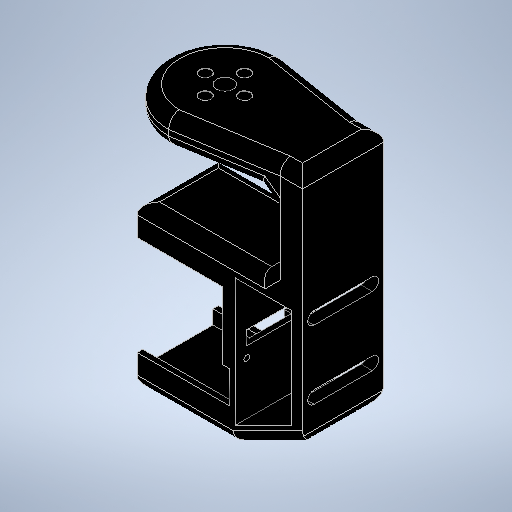
# Autodesk Inventor part: wahaczv6
Saved by Autodesk Inventor 2025.3 (Build 293356000, 356)
## iProperties
Created: 2026-04-05
Part Number: wahaczv6
Material: PCTG 20%
Document SubType Name: Modeling
Designer: ksawe
Density: 1.541 g/cm^3
Appearance: Anodized - Black
Mass: 108.544 g
Surface Area: 247.96 cm^2
Volume: 70.4373 cm^3
Author: ksawe
Autodesk Inventor part; units mm, degrees
ref_plane "YZ Plane" through (0, 0, 0) normal (1, 0, 0) x (0, 1, 0)
ref_plane "XZ Plane" through (0, 0, 0) normal (0, 1, 0) x (-1, 0, 0)
sketch "Sketch1" plane through (0, 0, 0) normal (0, 0, 1) x (1, 0, 0)
  line L0 (-59, 0) -> (-59, 6)
  line L1 (-59, 6) -> (-26, 6)
  line L2 (-26, 6) -> (-26, 51.5)
  line L3 (-26, 51.5) -> (-59, 51.5)
  line L4 (-59, 51.5) -> (-59, 57.5)
  line L5 (-59, 57.5) -> (-8, 57.5)
  line L6 (-8, 57.5) -> (-8, 95)
  line L7 (-8, 95) -> (0, 95)
  line L8 (-24, 51.5) -> (-4, 51.5)
  line L9 (-24, 51.5) -> (-24, 16)
  line L10 (-4, 51.5) -> (-4, 16)
  line L11 (-4, 16) -> (-24, 6)
  line L12 (-59, 0) -> (-24, 0)
  line L13 (-24, 0) -> (0, 12)
  line L14 (-24, 16) -> (-24, 6)
  line L15 (0, 95) -> (0, 12)
  point P0 (0, 0)
  dimension "d1" = 33
  dimension "d3" = 33
  dimension "d4" = 6
  dimension "d5" = 6
  dimension "d6" = 51
  dimension "d8" = 8
  dimension "d9" = 95
  dimension "d13" = 2
  dimension "d116" = 12
  dimension "d117" = 4
  dimension "d118" = 57.5
  constraints: 32 end point, 7 vertical, 5 vertical alignment, 4 horizontal, 4 horizontal alignment, 2 parallel, 2 perpendicular, 2 point on line
  measures "d1" distance of L0.end L1.end
  measures "d3" distance of L2.end L3.end
  measures "d4" distance of L3.end L4.end
  measures "d5" distance of L0.start L0.end
  measures "d6" distance of L4.end L5.end
  measures "d8" distance of L6.end L7.end
  measures "d9" distance of L7.end point (0, 0)
  measures "d13" distance between parallel lines of L9 L2
  measures "d116" vertical distance of L13.end L12.end
  measures "d117" distance between parallel lines of L15 L10
  measures "d118" distance between parallel lines of L12 L5
extrude "Extrusion1" add sketch "Sketch1" along normal mid plane 29
sketch "Sketch2" plane through (-8, 95, 14.5) normal (0, 1, 0) x (1, 0, 0)
  line L0 (0, 29) -> (0, 0) projected
  arc A0 (-34.2, 34.5) -> (-34.2, -5.5) centre (-34.2, 14.5) ccw
  line L1 (4, 29) -> (4, 0) projected
  line L2 (-34.2, 34.5) -> (0, 29)
  line L3 (8, 0) -> (0, 0) projected
  line L4 (0, 0) -> (-34.2, -5.5)
  circle A1 centre (-34.2, 14.5) radius 3
  circle A2 centre (-34.2, 21.5) radius 1.25
  circle A3 centre (-41.2, 14.5) radius 1.25
  circle A4 centre (-34.2, 7.5) radius 1.25
  circle A5 centre (-27.2, 14.5) radius 1.25
  point P0 (8, 14.5)
  point P1 (0, 14.5)
  point P2 (0, 14.5)
  dimension "d17" = 40
  dimension "d18" = 34.2
  dimension "d47" = 6
  dimension "d51" = 360
  dimension "d53" = 7
  dimension "d54" = 2.5
  constraints: 6 centre point, 4 end point, 2 midpoint, 2 point on circle, 2 vertical alignment, 1 coincident, 1 equal length, 1 horizontal alignment, 10 other
  measures "d17" diameter of A0
  measures "d18" distance of point (0, 14.5) A0.centre
  measures "d47" diameter of A1
  measures "d53" horizontal distance of A5.centre A2.centre
  measures "d54" diameter of A2
extrude "Extrusion2" add sketch "Sketch2" against normal blind 10 contours L0 L4 A0 L2 | A2 | A3 | A4 | A5
sketch "Sketch3" plane through (-26, 6, 14.5) normal (-1, 0, 0) x (0, 0, 1)
  line L0 (-29, 45.5) -> (0, 45.5) projected
  line L1 (-29, 0) -> (-29, 45.5) projected
  line L2 (0, 45.5) -> (0, 0) projected
  line L3 (-29, 0) -> (0, 0) construction
  line L4 (-14.5, 0) -> (-14.5, 45.5)
  line L5 (-29, 45.5) -> (0, 45.5) projected
  line L6 (-24.5, 40.5) -> (-4.5, 40.5)
  line L7 (-25.1, 27.5) -> (-3.9, 27.5)
  line L8 (-29, 45.5) -> (0, 45.5) construction
  line L9 (-25.1, 27.5) -> (-25.1, 22.5)
  line L10 (-25.1, 22.5) -> (-26.1, 22.5)
  line L11 (-26.1, 22.5) -> (-26.1, 27.5)
  line L12 (-26.1, 27.5) -> (-25.1, 27.5)
  line L13 (-3.9, 27.5) -> (-3.9, 22.5)
  line L14 (-3.9, 22.5) -> (-2.9, 22.5)
  line L15 (-2.9, 22.5) -> (-2.9, 27.5)
  line L16 (-2.9, 27.5) -> (-3.9, 27.5)
  line L17 (-25.1, 22.5) -> (-3.9, 22.5)
  line L18 (-29, 45.5) -> (-29, 0) projected
  line L19 (-22, 22.5) -> (-22, 20.5)
  line L20 (-24.5, 16.5) -> (-29, 16.5)
  line L21 (-24.5, 40.5) -> (-24.5, 27.5)
  line L22 (-7, 20.5) -> (-4.5, 16.5)
  line L23 (-4.5, 16.5) -> (0, 16.5)
  line L24 (-4.5, 40.5) -> (-4.5, 27.5)
  line L25 (-7, 22.5) -> (-7, 20.5)
  circle A0 centre (-24.89, 43.14) radius 1.05
  circle A1 centre (-24.89, 18.69) radius 1.05
  circle A2 centre (-4.11, 43.14) radius 1.05
  circle A3 centre (-4.11, 18.69) radius 1.05
  line L26 (-22, 20.5) -> (-24.5, 16.5)
  point P0 (-14.5, -6)
  point P1 (-14.5, 40.5)
  point P2 (-14.5, 27.5)
  point P3 (-29, 14)
  point P4 (-14.5, 40.5)
  point P5 (-14.5, 45.5)
  point P6 (-14.5, 27.5)
  point P7 (-14.5, 22.5)
  dimension "d22" = 5
  dimension "d25" = 2
  dimension "d26" = 5
  dimension "d30" = 13
  dimension "d33" = 2.1
  dimension "d34" = 2.1
  dimension "d35" = 24.45
  dimension "d37" = 2.36
  dimension "d40" = 6
  dimension "d44" = 4.11
  dimension "d46" = 2.5
  dimension "d83" = 2.9
  dimension "d84" = 1.6
  dimension "d85" = 1
  dimension "d86" = 20
  constraints: 40 end point, 10 symmetric about line, 6 midpoint, 5 perpendicular, 4 centre point, 4 vertical alignment, 2 horizontal, 2 point on line, 2 vertical, 2 other
  measures "d22" distance between parallel lines of L0 L6
  measures "d25" distance of L19.start L19.end
  measures "d26" distance of L10.end L11.end
  measures "d30" distance of L6.start L21.end
  measures "d33" diameter of A0
  measures "d34" diameter of A1
  measures "d35" distance of A0.centre A1.centre
  measures "d37" distance from line of L0 A0.centre
  measures "d40" distance between parallel lines of L20 L17
  measures "d44" distance from line of L18 A1.centre
  measures "d46" horizontal distance of L19.end L20.start
  measures "d83" distance between parallel lines of L1 L11
  measures "d84" distance from line of L11.end L21
  measures "d85" distance between parallel lines of L9 L11
  measures "d86" distance of L6.start L6.end
extrude "Extrusion3" add sketch "Sketch3" along normal blind 2.5 contours L0 L4 L6 L21 L7 L12 L11 L10 L17 L19 L26 L20 L1 | L0 L2 L23 L22 L25 L17 L14 L15 L16 L7 L24 L6 L4 | L9 L10 L11 L12 | L16 L15 L14 L13
extrude "Extrusion4" cut sketch "Sketch3" against normal up to surface (2 mm away) contours L7 L13 L17 L4 | L4 L17 L9 L7 | A0 | A1 | A2 | A3
hole "Hole1" at (-49.2, 95, 0) at (-42.2, 95, -7) at (-35.2, 95, 0) at (-42.2, 95, 7) direction (0, -1, 0) diameter 4 depth 7 countersink diameter 4.2 countersink angle 90
ref_plane "Work Plane1" through (-26, 28.5, 0) normal (0, 1, 0) x (1, 0, 0)
sketch "Sketch6" plane through (-59, 6, 14.5) normal (0, 1, 0) x (1, 0, 0)
  line L0 (33, 29) -> (33, 0) projected
  line L1 (33, 2) -> (0, 2)
  line L2 (33, 0) -> (0, 0) projected
  line L3 (0, 29) -> (0, 0) projected
  line L4 (33, 27) -> (0, 27)
  line L5 (0, 29) -> (33, 29) projected
  point P0 (59, 14.5)
  dimension "d74" = 2
  dimension "d75" = 2
  constraints: 4 end point, 3 point on line, 1 parallel, 1 perpendicular
  measures "d74" distance between parallel lines of L2 L1
  measures "d75" distance between parallel lines of L5 L4
extrude "Extrusion7" add sketch "Sketch6" along normal blind 5 contours L0 L4 L3 L5 | L0 L2 L3 L1
sketch "Sketch7" plane through (-59, 51.5, -14.5) normal (0, -1, 0) x (1, 0, 0)
  line L0 (0, 0) -> (0, 29) projected
  line L1 (0, 29) -> (30.5, 29) projected
  line L2 (30.5, 0) -> (0, 0) projected
  line L3 (30.5, 0) -> (30.5, 29) projected
  line L4 (30.5, 2) -> (0, 2)
  line L5 (30.5, 27) -> (0, 27)
  point P0 (59, 14.5)
  dimension "d78" = 2
  dimension "d79" = 2
  constraints: 4 end point, 4 point on line, 2 perpendicular, 1 parallel
  measures "d78" distance between parallel lines of L1 L5
  measures "d79" distance between parallel lines of L4 L2
extrude "Extrusion8" add sketch "Sketch7" along normal blind 5 contours L0 L4 L3 L2 | L0 L1 L3 L5
sketch "Sketch10" plane through (0, 12, 14.5) normal (1, 0, 0) x (0, 0, -1)
  circle A0 centre (4.11, 12.69) radius 1.05 projected
  circle A1 centre (24.89, 37.14) radius 1.05 projected
  circle A2 centre (24.89, 12.69) radius 1.05 projected
  line L0 (29, 39.5) -> (0, 39.5) projected
  circle A3 centre (4.11, 37.14) radius 1.05 projected
  line L1 (4.11, 37.14) -> (24.89, 37.14) construction
  line L2 (4.5, 34.5) -> (24.5, 34.5) projected
  line L3 (4.11, 34.89) -> (24.89, 34.89)
  line L4 (24.89, 39.39) -> (4.11, 39.39)
  arc A4 (4.11, 39.39) -> (4.11, 34.89) centre (4.11, 37.14) ccw
  arc A5 (24.89, 34.89) -> (24.89, 39.39) centre (24.89, 37.14) ccw
  line L5 (4.11, 12.69) -> (24.89, 12.69) construction
  line L6 (4.11, 10.44) -> (24.89, 10.44)
  line L7 (24.89, 14.94) -> (4.11, 14.94)
  arc A6 (4.11, 14.94) -> (4.11, 10.44) centre (4.11, 12.69) ccw
  arc A7 (24.89, 10.44) -> (24.89, 14.94) centre (24.89, 12.69) ccw
  point P0 (14.5, -12)
  point P1 (26, 39.5)
  point P2 (3, 39.5)
  point P3 (14.5, 37.14)
  point P4 (14.5, 12.69)
  dimension "d123" = 4.5
  dimension "d124" = 4.5
  constraints: 16 end point, 8 point on circle, 8 tangent, 4 centre point, 4 parallel, 2 midpoint
  measures "d123" diameter of A5
  measures "d124" diameter of A7
extrude "Extrusion12" cut sketch "Sketch10" against normal up to surface (4 mm away) contours A0 | A1 | A2 | A3 | A4 L4 A5 L3 | A6 L7 A7 L6
chamfer "Chamfer7" distance 7 angle 45 2 edges at (-8, 57.5, 0) (-8, 85, 0)
fillet "Fillet8" radius 4 22 edges at (-62.2, 95, 0) (-25.1, 95, 17.25) (-4, 95, 14.5) (0, 95, 0) (0, 12, 0) (-12, 6, 14.5) (-41.5, 0, 14.5) (-41.5, 0, -14.5) (-12, 6, -14.5) (-59, 0, 0) (-37, 57.5, 14.5) (-37, 57.5, -14.5) (-11.5, 61, 14.5) (-11.5, 61, -14.5) (-11.5, 81.5, -15.0629) (-28.6, 85, -17.8129) (-62.2, 85, 0) (-28.6, 85, 17.8129) (-11.5, 81.5, 15.0629) (-59, 57.5, 0) (-25.1, 95, -17.25) (-4, 95, -14.5)
body "Solid1"
